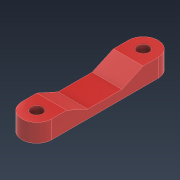
# Autodesk Inventor part: CH_01_0052_bracket_mount
Saved by Autodesk Inventor 2022.3 (Build 263350030, 350C)
## iProperties
Created: 2022-08-31
Part Number: CH_01_0052_bracket_mount
Material: Generic
Document SubType Name: Modeling
Designer: Tomasz Krakowski
Density: 1 g/cm^3
Appearance: Orange-Red
Author: Tomasz Krakowski
Autodesk Inventor part; units mm, degrees
ref_plane "YZ Plane" through (0, 0, 0) normal (1, 0, 0) x (0, 1, 0)
ref_plane "XZ Plane" through (0, 0, 0) normal (0, 1, 0) x (-1, 0, 0)
ref_plane "XY Plane" through (0, 0, 0) normal (0, 0, 1) x (1, 0, 0)
sketch "Sketch1" plane through (0, 0, 0) normal (0, 1, 0) x (-1, 0, 0)
  line L0 (-7, 32) -> (7, 32)
  line L1 (7, 32) -> (7, -32)
  line L2 (7, -32) -> (-7, -32)
  line L3 (-7, -32) -> (-7, 32)
  line L4 (-7, 32) -> (7, -32) construction
  line L5 (7, 32) -> (-7, -32) construction
  circle A0 centre (0, 25) radius 2.75
  circle A1 centre (0, -25) radius 2.75
  line L6 (0, 25) -> (0, 0) construction
  line L7 (0, 0) -> (0, -25) construction
  dimension "d0" = 5.5
  dimension "d1" = 50
  dimension "d3" = 7
  dimension "d4" = 7
  constraints: 16 end point, 2 centre point, 2 midpoint, 2 parallel, 2 vertical, 1 collinear, 1 equal radius, 1 horizontal, 1 perpendicular
  measures "d0" diameter of A0
  measures "d1" distance of L7.end L6.start
  measures "d3" distance from line of L0 L6.start
  measures "d4" distance from line of L6.start L1
extrude "Extrusion1" add sketch "Sketch1" along normal blind 8.5
sketch "Sketch2" plane through (7, 0, 32) normal (1, 0, 0) x (0, 0, -1)
  line L0 (64, 8.5) -> (0, 8.5) construction
  line L1 (14, 8.5) -> (24, 4)
  line L2 (24, 4) -> (32, 4)
  line L3 (32, 4) -> (32, 0) construction
  line L4 (50, 8.5) -> (40, 4)
  line L5 (40, 4) -> (32, 4)
  line L6 (14, 8.5) -> (50, 8.5)
  line L7 (0, 0) -> (64, 0) projected
  line L8 (4.25, 8.5) -> (9.75, 8.5) projected
  point P0 (7, 8.5)
  dimension "d7" = 4
  dimension "d8" = 7
  dimension "d9" = 10
  constraints: 12 end point, 2 symmetric about line, 1 collinear, 1 midpoint, 1 parallel, 1 perpendicular, 1 point on line
  measures "d7" distance between parallel lines of L7 L2
  measures "d8" distance of L1.start point (7, 8.5)
  measures "d9" horizontal distance of L1.start L1.end
extrude "Extrusion2" cut sketch "Sketch2" against normal through all
fillet "Fillet1" radius 7 4 edges at (7, 4.25, 32) (-7, 4.25, 32) (-7, 4.25, -32) (7, 4.25, -32)
body "Solid1"
